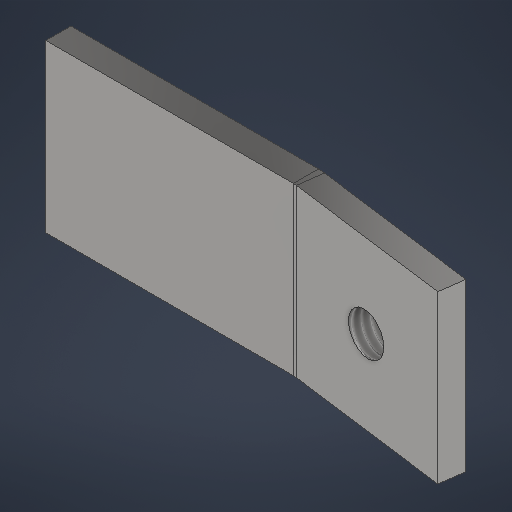
# Autodesk Inventor part: Pressure platform
Saved by Autodesk Inventor 2026.3 (Build 303398000, 398)
## iProperties
Created: 2026-08-04
Part Number: Pressure platform
Material: Generic
Document SubType Name: Sheet Metal
Designer: matot
Density: 1 g/cm^3
Sheet Metal Rule: Default_mm
Appearance: Default
Author: matot
Autodesk Inventor part; units mm, degrees
ref_plane "YZ Plane" through (0, 0, 0) normal (1, 0, 0) x (0, 1, 0)
ref_plane "XZ Plane" through (0, 0, 0) normal (0, 1, 0) x (-1, 0, 0)
ref_plane "XY Plane" through (0, 0, 0) normal (0, 0, 1) x (1, 0, 0)
sketch "Sketch1" plane through (0, 0, 0) normal (0, 0, 1) x (1, 0, 0)
  line L0 (-18, 8) -> (32, 8)
  line L1 (32, 8) -> (32, -12)
  line L2 (32, -12) -> (-18, -12)
  line L3 (-18, -12) -> (-18, 8)
  point P0 (0, 0)
  dimension "d0" = 50
  dimension "d1" = 20
  measures "d0" distance of L0.start L0.end
  measures "d1" distance of L2.end L0.start
extrude "Plate1" add sketch "Sketch1" along normal blind 3
sketch "Sketch2" plane through (0, 0, 3) normal (0, 0, 1) x (1, 0, 0)
  line L0 (32, 8) -> (-18, 8) projected
  line L1 (12, 8) -> (12, -12)
  line L2 (-18, -12) -> (32, -12) projected
  line L3 (32, -12) -> (-18, -12) projected
  line L4 (32, 8) -> (32, -12) projected
  point P0 (0, 0)
  dimension "d3" = 20
  constraints: 2 end point, 2 point on line, 1 perpendicular, 1 vertical
  measures "d3" distance between parallel lines of L4 L1
fold "Fold1" angle 7.5 bend radius 3 thickness 3 k factor 0.44 line from (12, 8, 3) to (12, -12, 3) line at bend centre moving side (1, 0, 0) folds toward (0, 0, 1)
sketch "Sketch4" plane through (31.6574, -12, 5.5993) normal (-0.1305262, 0, 0.9914449) x (0.9914449, 0, 0.1305262)
  line L0 (0, 20) -> (0, 0) projected
  line L1 (0, 0) -> (-19.7173, 0) projected
  point P0 (-32.1174, 12)
  point P1 (-10, 10)
  point P2 (0, 10)
  dimension "d10" = 10
  dimension "d11" = 10
  constraints: 1 midpoint
  measures "d10" distance of point (0, 10) point (-10, 10)
  measures "d11" distance from line of L1 point (-10, 10)
hole "Hole1" at (21.743, -2, 4.294) direction (0.1305262, 0, -0.9914449) diameter 4.917 end through all thread size "M6x1" class "6H" standard "ISO Metric profile"
equation "\"d2\" = Thickness"
equation "\"d4\" = BendReliefWidth"
equation "\"d5\" = BendReliefDepth"
equation "\"d6\" = MinimumRemnant"
equation "\"d7\" = TransitionRadius"
equation "\"d9\" = BendRadius"
equation "\"d17\" = Thickness"
equation "\"BendRadius\" = Thickness"
equation "\"BendReliefWidth\" = Thickness"
equation "\"BendReliefDepth\" = 0.5 * Thickness"
equation "\"CornerReliefSize\" = 4 * Thickness"
equation "\"MinimumRemnant\" = 2 * Thickness"
equation "\"TransitionRadius\" = BendRadius"
equation "\"JacobiRadiusSize\" = BendRadius"
equation "\"GapSize\" = Thickness"
equation "\"Thickness\" = 3"
body "Solid1"
